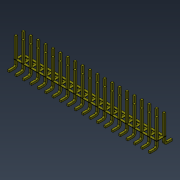
# Autodesk Inventor part: T-1S6-16(-01-20-DV)
Saved by Autodesk Inventor 2022.1 (Build 261234020, 234B)
## iProperties
Created: 2015-08-01
Part Number: T-1S6-16(-01-20-DV)
Catalog Web Link: www.cadenas.de
Description: TSM Series Terminal-TSM Series - (2,54 mm) .100" Surface Mount Terminal .025" Square Post Header
Vendor: SAMTEC
Document SubType Name: Modeling
Designer: PARTuser1
Manufacturer: SAMTEC
Mass: 0.198411 g
Surface Area: 13.9569 cm^2
Volume: 0.198411 cm^3
Density: 1 g/cm^3
Material: Allgemein
Appearance: PSOLRGB-255-255-0
Category: PARTsolutions
Company: SAMTEC
PSOL_IDENT_0: {$CADENAS_DATA\23d-libs\samtec\modelling\tsm\parts\tsm_terminal.prj},210 {VTYP=3D},{NB=T-1S6-16(-01-
PSOL_IDENT_1: 20-DV)},{LINA=T-1S6-16(-01-20-DV)},{NN=TSM Series Terminal},{DATE=20.05.2015 06:36:02},{GEOMDATE=20.
PSOL_IDENT_2: 05.2015 06:36:00},{VERSION=},{LINEID=10},{LINESUBID=-1},{WBVAR=POS,LS,ROW,POLOPT}  {NB=T-1S6-16(-01-
PSOL_IDENT_3: 20-DV)},{LINA=T-1S6-16(-01-20-DV)},{KT=DUMMY},{PN=T-1S6-16},{POS=20},{LS=-01},{LSALG= '-01','-01','-
PSOL_IDENT_4: 02','-02','-03','-03','-04','-04' ,'-05','-05 (Non-standard option -  Please contact SAMTEC)' },{ROW=
PSOL_IDENT_5: -DV},{ROWALG= '-SV','-SV - Single Vertical', '-SH','-SH - Single Horizontal', '-DV' ,'-DV - Double V
PSOL_IDENT_6: ertical' ,'-DV-S' ,'-DV-S - Double Vertical Molded End Shrouds (Non-standard option -  Please contac
PSOL_IDENT_7: t SAMTEC)', '-DH', '-DH - Double Horizontal' ,  '-MT','-MT - Mixed Technology','-EM','-EM - Edge Mou
PSOL_IDENT_8: nt', '-TM','-TM - Triple Mixed Technology'  },{POLOPT=},{POLOPTALG= '','Not Selected','001','001','0
PSOL_IDENT_9: 02','002','003','003','004','004','005','005','006','006','007','007','008','008','009','009','010','
PSOL_IDENT_10: 010','011','011','012','012','013','013','014','014','015','015','016','016','017','017','018','018'
PSOL_IDENT_11: ,'019','019','020','020','021','021','022','022','023','023','024','024','025','025','026','026','02
PSOL_IDENT_12: 7','027','028','028','029','029','030','030','031','031','032','032','033','033','034','034','035','
PSOL_IDENT_13: 035','036','036','037','037','038','038','039','039','040','040' },{POLOPTMAX=480},{POLOPTMAX2='001'
PSOL_IDENT_14: ,'001','002','002','003','003','004','004','005','005','006','006','007','007','008','008','009','00
PSOL_IDENT_15: 9','010','010','011','011','012','012','013','013','014','014','015','015','016','016','017','017','
PSOL_IDENT_16: 018','018','019','019','020','020','021','021','022','022','023','023','024','024','025','025','026'
PSOL_IDENT_17: ,'026','027','027','028','028','029','029','030','030','031','031','032','032','033','033','034','03
PSOL_IDENT_18: 4','035','035','036','036','037','037','038','038','039','039','040','040'},{POLARIZE='001','001','0
PSOL_IDENT_19: 02','002','003','003','004','004','005','005','006','006','007','007','008','008','009','009','010','
PSOL_IDENT_20: 010','011','011','012','012','013','013','014','014','015','015','016','016','017','017','018','018'
PSOL_IDENT_21: ,'019','019','020','020','021','021','022','022','023','023','024','024','025','025','026','026','02
PSOL_IDENT_22: 7','027','028','028','029','029','030','030','031','031','032','032','033','033','034','034','035','
PSOL_IDENT_23: 035','036','036','037','037','038','038','039','039','040','040','041','041','042','042','043','043'
PSOL_IDENT_24: ,'044','044','045','045','046','046','047','047','048','048','049','049','050','050','051','051','05
PSOL_IDENT_25: 2','052','053','053','054','054','055','055','056','056','057','057','058','058','059','059','060','
PSOL_IDENT_26: 060','061','061','062','062','063','063','064','064','065','065','066','066','067','067','068','068'
PSOL_IDENT_27: ,'069','069','070','070','071','071','072','072','073','073','074','074','075','075','076','076','07
PSOL_IDENT_28: 7','077','078','078','079','079','080','080','081','081','082','082','083','083','084','084','085','
PSOL_IDENT_29: 085','086','086','087','087','088','088','089','089','090','090','091','091','092','092','093','093'
PSOL_IDENT_30: ,'094','094','095','095','096','096','097','097','098','098','099','099','100','100','101','101','10
PSOL_IDENT_31: 2','102','103','103','104','104','105','105','106','106','107','107','108','108','109','109','110','
PSOL_IDENT_32: 110','111','111','112','112','113','113','114','114','115','115','116','116','117','117','118','118'
PSOL_IDENT_33: ,'119','119','120','120','121','121','122','122','123','123','124','124','125','125','126','126','12
PSOL_IDENT_34: 7','127','128','128','129','129','130','130','131','131','132','132','133','133','134','134','135','
PSOL_IDENT_35: 135','136','136','137','137','138','138','139','139','140','140','141','141','142','142','143','143'
PSOL_IDENT_36: ,'144','144','145','145','146','146','147','147','148','148','149','149','150','150'},{POLOPTPN=},{P
PSOL_IDENT_37: OLOPTATOF=0},{BSH=0.230},{CSH=0.180},{BSV=0.230},{DMAXSV=0.208},{AEM=0.230},{POLOE=0},{CDHMT=0.230},
PSOL_IDENT_38: {BDVTM=0.23000},{CDV=0.30300},{POLTM=0}
NN: TSM Series Terminal
NT: TSM Series - (2,54 mm) .100" Surface Mount Terminal .025" Square Post Header
NB: T-1S6-16(-01-20-DV)
NBSYN: $PN.($LS.-$POS.$ROW.$POLOPT.)
LINA: T-1S6-16(-01-20-DV)
POS: 20
LS: -01
ROW: -DV - Double Vertical
POLOPT: Not Selected
SUPPLIER: SAMTEC
ARTICLENO: T-1S6-16(-01-20-DV)
BOMINFO: T-1S6-16(-01-20-DV)
CREATOR: CADENAS GmbH
Title: T-1S6-16(-01-20-DV)
Author: Cadenas PARTsolutions
Comments: TSM Series - (2,54 mm) .100" Surface Mount Terminal .025" Square Post Header
Autodesk Inventor part; units mm, degrees
sketch "Sketch_1" plane through (0, 0, 0) normal (1, 0, 0) x (0, 1, 0)
  line L0 (0.635, 2.5781) -> (0, 2.5781)
  line L1 (0, 2.5781) -> (0, 0.6985)
  arc A0 (0, 0.6985) -> (1.016, -0.3175) centre (1.016, 0.6985) ccw
  line L2 (1.016, -0.3175) -> (9.652, -0.3175)
  line L3 (9.652, -0.3175) -> (9.652, 0.3175)
  line L4 (9.652, 0.3175) -> (1.143, 0.3175)
  arc A1 (0.635, 0.8255) -> (1.143, 0.3175) centre (1.143, 0.8255) ccw
  line L5 (0.635, 0.8255) -> (0.635, 2.5781)
  constraints: 12 end point, 4 point on circle, 2 centre point
extrude "Extrusion1" add sketch "Sketch_1" along normal mid plane 48.895
sketch "Sketch_4" plane through (0, 2.54, 0) normal (0, 1, 0) x (1, 0, 0)
  line L0 (-24.4983, 2.9083) -> (-24.4983, -0.3683)
  line L1 (-24.4983, -0.3683) -> (24.4983, -0.3683)
  line L2 (24.4983, -0.3683) -> (24.4983, 2.9083)
  line L3 (24.4983, 2.9083) -> (-24.4983, 2.9083)
  line L4 (21.9583, 2.1717) -> (21.9583, 0.3683)
  line L5 (21.9583, 0.3683) -> (23.7617, 0.3683)
  line L6 (23.7617, 0.3683) -> (23.7617, 2.1717)
  line L7 (23.7617, 2.1717) -> (21.9583, 2.1717)
  line L8 (19.4183, 2.1717) -> (19.4183, 0.3683)
  line L9 (19.4183, 0.3683) -> (21.2217, 0.3683)
  line L10 (21.2217, 0.3683) -> (21.2217, 2.1717)
  line L11 (21.2217, 2.1717) -> (19.4183, 2.1717)
  line L12 (16.8783, 2.1717) -> (16.8783, 0.3683)
  line L13 (16.8783, 0.3683) -> (18.6817, 0.3683)
  line L14 (18.6817, 0.3683) -> (18.6817, 2.1717)
  line L15 (18.6817, 2.1717) -> (16.8783, 2.1717)
  line L16 (14.3383, 2.1717) -> (14.3383, 0.3683)
  line L17 (14.3383, 0.3683) -> (16.1417, 0.3683)
  line L18 (16.1417, 0.3683) -> (16.1417, 2.1717)
  line L19 (16.1417, 2.1717) -> (14.3383, 2.1717)
  line L20 (11.7983, 2.1717) -> (11.7983, 0.3683)
  line L21 (11.7983, 0.3683) -> (13.6017, 0.3683)
  line L22 (13.6017, 0.3683) -> (13.6017, 2.1717)
  line L23 (13.6017, 2.1717) -> (11.7983, 2.1717)
  line L24 (9.2583, 2.1717) -> (9.2583, 0.3683)
  line L25 (9.2583, 0.3683) -> (11.0617, 0.3683)
  line L26 (11.0617, 0.3683) -> (11.0617, 2.1717)
  line L27 (11.0617, 2.1717) -> (9.2583, 2.1717)
  line L28 (6.7183, 2.1717) -> (6.7183, 0.3683)
  line L29 (6.7183, 0.3683) -> (8.5217, 0.3683)
  line L30 (8.5217, 0.3683) -> (8.5217, 2.1717)
  line L31 (8.5217, 2.1717) -> (6.7183, 2.1717)
  line L32 (4.1783, 2.1717) -> (4.1783, 0.3683)
  line L33 (4.1783, 0.3683) -> (5.9817, 0.3683)
  line L34 (5.9817, 0.3683) -> (5.9817, 2.1717)
  line L35 (5.9817, 2.1717) -> (4.1783, 2.1717)
  line L36 (1.6383, 2.1717) -> (1.6383, 0.3683)
  line L37 (1.6383, 0.3683) -> (3.4417, 0.3683)
  line L38 (3.4417, 0.3683) -> (3.4417, 2.1717)
  line L39 (3.4417, 2.1717) -> (1.6383, 2.1717)
  line L40 (-0.9017, 2.1717) -> (-0.9017, 0.3683)
  line L41 (-0.9017, 0.3683) -> (0.9017, 0.3683)
  line L42 (0.9017, 0.3683) -> (0.9017, 2.1717)
  line L43 (0.9017, 2.1717) -> (-0.9017, 2.1717)
  line L44 (-3.4417, 2.1717) -> (-3.4417, 0.3683)
  line L45 (-3.4417, 0.3683) -> (-1.6383, 0.3683)
  line L46 (-1.6383, 0.3683) -> (-1.6383, 2.1717)
  line L47 (-1.6383, 2.1717) -> (-3.4417, 2.1717)
  line L48 (-5.9817, 2.1717) -> (-5.9817, 0.3683)
  line L49 (-5.9817, 0.3683) -> (-4.1783, 0.3683)
  line L50 (-4.1783, 0.3683) -> (-4.1783, 2.1717)
  line L51 (-4.1783, 2.1717) -> (-5.9817, 2.1717)
  line L52 (-8.5217, 2.1717) -> (-8.5217, 0.3683)
  line L53 (-8.5217, 0.3683) -> (-6.7183, 0.3683)
  line L54 (-6.7183, 0.3683) -> (-6.7183, 2.1717)
  line L55 (-6.7183, 2.1717) -> (-8.5217, 2.1717)
  line L56 (-11.0617, 2.1717) -> (-11.0617, 0.3683)
  line L57 (-11.0617, 0.3683) -> (-9.2583, 0.3683)
  line L58 (-9.2583, 0.3683) -> (-9.2583, 2.1717)
  line L59 (-9.2583, 2.1717) -> (-11.0617, 2.1717)
  line L60 (-13.6017, 2.1717) -> (-13.6017, 0.3683)
  line L61 (-13.6017, 0.3683) -> (-11.7983, 0.3683)
  line L62 (-11.7983, 0.3683) -> (-11.7983, 2.1717)
  line L63 (-11.7983, 2.1717) -> (-13.6017, 2.1717)
  line L64 (-16.1417, 2.1717) -> (-16.1417, 0.3683)
  line L65 (-16.1417, 0.3683) -> (-14.3383, 0.3683)
  line L66 (-14.3383, 0.3683) -> (-14.3383, 2.1717)
  line L67 (-14.3383, 2.1717) -> (-16.1417, 2.1717)
  line L68 (-18.6817, 2.1717) -> (-18.6817, 0.3683)
  line L69 (-18.6817, 0.3683) -> (-16.8783, 0.3683)
  line L70 (-16.8783, 0.3683) -> (-16.8783, 2.1717)
  line L71 (-16.8783, 2.1717) -> (-18.6817, 2.1717)
  line L72 (-21.2217, 2.1717) -> (-21.2217, 0.3683)
  line L73 (-21.2217, 0.3683) -> (-19.4183, 0.3683)
  line L74 (-19.4183, 0.3683) -> (-19.4183, 2.1717)
  line L75 (-19.4183, 2.1717) -> (-21.2217, 2.1717)
  line L76 (-23.7617, 2.1717) -> (-23.7617, 0.3683)
  line L77 (-23.7617, 0.3683) -> (-21.9583, 0.3683)
  line L78 (-21.9583, 0.3683) -> (-21.9583, 2.1717)
  line L79 (-21.9583, 2.1717) -> (-23.7617, 2.1717)
  constraints: 160 end point
extrude "Extrusion2" add sketch "Sketch_4" along normal blind 0.127
sketch "Sketch_5" plane through (0, 0, 0) normal (1, 0, 0) x (0, 1, 0)
  arc A0 (1.016, -2.2225) -> (0, -3.2385) centre (1.016, -3.2385) ccw
  line L0 (0, -3.2385) -> (0, -5.1181)
  line L1 (0, -5.1181) -> (0.635, -5.1181)
  line L2 (0.635, -5.1181) -> (0.635, -3.3655)
  arc A1 (1.143, -2.8575) -> (0.635, -3.3655) centre (1.143, -3.3655) ccw
  line L3 (1.143, -2.8575) -> (9.652, -2.8575)
  line L4 (9.652, -2.8575) -> (9.652, -2.2225)
  line L5 (9.652, -2.2225) -> (1.016, -2.2225)
  constraints: 12 end point, 4 point on circle, 2 centre point
extrude "Extrusion3" add sketch "Sketch_5" along normal mid plane 48.895
sketch "Sketch_7" plane through (0, 0, 0) normal (0, 0, 1) x (1, 0, 0)
  line L0 (-23.8125, 18.0594) -> (-23.8125, 2.667)
  line L1 (-23.8125, 2.667) -> (-21.9075, 2.667)
  line L2 (-21.9075, 2.667) -> (-21.9075, 15.3924)
  line L3 (-21.9075, 15.3924) -> (-21.2725, 15.3924)
  line L4 (-21.2725, 15.3924) -> (-21.2725, 2.667)
  line L5 (-21.2725, 2.667) -> (-19.3675, 2.667)
  line L6 (-19.3675, 2.667) -> (-19.3675, 15.3924)
  line L7 (-19.3675, 15.3924) -> (-18.7325, 15.3924)
  line L8 (-18.7325, 15.3924) -> (-18.7325, 2.667)
  line L9 (-18.7325, 2.667) -> (-16.8275, 2.667)
  line L10 (-16.8275, 2.667) -> (-16.8275, 15.3924)
  line L11 (-16.8275, 15.3924) -> (-16.1925, 15.3924)
  line L12 (-16.1925, 15.3924) -> (-16.1925, 2.667)
  line L13 (-16.1925, 2.667) -> (-14.2875, 2.667)
  line L14 (-14.2875, 2.667) -> (-14.2875, 15.3924)
  line L15 (-14.2875, 15.3924) -> (-13.6525, 15.3924)
  line L16 (-13.6525, 15.3924) -> (-13.6525, 2.667)
  line L17 (-13.6525, 2.667) -> (-11.7475, 2.667)
  line L18 (-11.7475, 2.667) -> (-11.7475, 15.3924)
  line L19 (-11.7475, 15.3924) -> (-11.1125, 15.3924)
  line L20 (-11.1125, 15.3924) -> (-11.1125, 2.667)
  line L21 (-11.1125, 2.667) -> (-9.2075, 2.667)
  line L22 (-9.2075, 2.667) -> (-9.2075, 15.3924)
  line L23 (-9.2075, 15.3924) -> (-8.5725, 15.3924)
  line L24 (-8.5725, 15.3924) -> (-8.5725, 2.667)
  line L25 (-8.5725, 2.667) -> (-6.6675, 2.667)
  line L26 (-6.6675, 2.667) -> (-6.6675, 15.3924)
  line L27 (-6.6675, 15.3924) -> (-6.0325, 15.3924)
  line L28 (-6.0325, 15.3924) -> (-6.0325, 2.667)
  line L29 (-6.0325, 2.667) -> (-4.1275, 2.667)
  line L30 (-4.1275, 2.667) -> (-4.1275, 15.3924)
  line L31 (-4.1275, 15.3924) -> (-3.4925, 15.3924)
  line L32 (-3.4925, 15.3924) -> (-3.4925, 2.667)
  line L33 (-3.4925, 2.667) -> (-1.5875, 2.667)
  line L34 (-1.5875, 2.667) -> (-1.5875, 15.3924)
  line L35 (-1.5875, 15.3924) -> (-0.9525, 15.3924)
  line L36 (-0.9525, 15.3924) -> (-0.9525, 2.667)
  line L37 (-0.9525, 2.667) -> (0.9525, 2.667)
  line L38 (0.9525, 2.667) -> (0.9525, 15.3924)
  line L39 (0.9525, 15.3924) -> (1.5875, 15.3924)
  line L40 (1.5875, 15.3924) -> (1.5875, 2.667)
  line L41 (1.5875, 2.667) -> (3.4925, 2.667)
  line L42 (3.4925, 2.667) -> (3.4925, 15.3924)
  line L43 (3.4925, 15.3924) -> (4.1275, 15.3924)
  line L44 (4.1275, 15.3924) -> (4.1275, 2.667)
  line L45 (4.1275, 2.667) -> (6.0325, 2.667)
  line L46 (6.0325, 2.667) -> (6.0325, 15.3924)
  line L47 (6.0325, 15.3924) -> (6.6675, 15.3924)
  line L48 (6.6675, 15.3924) -> (6.6675, 2.667)
  line L49 (6.6675, 2.667) -> (8.5725, 2.667)
  line L50 (8.5725, 2.667) -> (8.5725, 15.3924)
  line L51 (8.5725, 15.3924) -> (9.2075, 15.3924)
  line L52 (9.2075, 15.3924) -> (9.2075, 2.667)
  line L53 (9.2075, 2.667) -> (11.1125, 2.667)
  line L54 (11.1125, 2.667) -> (11.1125, 15.3924)
  line L55 (11.1125, 15.3924) -> (11.7475, 15.3924)
  line L56 (11.7475, 15.3924) -> (11.7475, 2.667)
  line L57 (11.7475, 2.667) -> (13.6525, 2.667)
  line L58 (13.6525, 2.667) -> (13.6525, 15.3924)
  line L59 (13.6525, 15.3924) -> (14.2875, 15.3924)
  line L60 (14.2875, 15.3924) -> (14.2875, 2.667)
  line L61 (14.2875, 2.667) -> (16.1925, 2.667)
  line L62 (16.1925, 2.667) -> (16.1925, 15.3924)
  line L63 (16.1925, 15.3924) -> (16.8275, 15.3924)
  line L64 (16.8275, 15.3924) -> (16.8275, 2.667)
  line L65 (16.8275, 2.667) -> (18.7325, 2.667)
  line L66 (18.7325, 2.667) -> (18.7325, 15.3924)
  line L67 (18.7325, 15.3924) -> (19.3675, 15.3924)
  line L68 (19.3675, 15.3924) -> (19.3675, 2.667)
  line L69 (19.3675, 2.667) -> (21.2725, 2.667)
  line L70 (21.2725, 2.667) -> (21.2725, 15.3924)
  line L71 (21.2725, 15.3924) -> (21.9075, 15.3924)
  line L72 (21.9075, 15.3924) -> (21.9075, 2.667)
  line L73 (21.9075, 2.667) -> (23.8125, 2.667)
  line L74 (23.8125, 2.667) -> (23.8125, 18.0594)
  line L75 (23.8125, 18.0594) -> (-23.8125, 18.0594)
  constraints: 152 end point
extrude "Extrusion4" cut sketch "Sketch_7" along normal mid plane 10.16
sketch "Sketch_8" plane through (0, 0, 0) normal (0, 0, 1) x (1, 0, 0)
  line L0 (-23.8125, -12.8524) -> (23.8125, -12.8524)
  line L1 (23.8125, -12.8524) -> (23.8125, 2.54)
  line L2 (23.8125, 2.54) -> (21.9075, 2.54)
  line L3 (21.9075, 2.54) -> (21.9075, -12.5984)
  line L4 (21.9075, -12.5984) -> (21.2725, -12.5984)
  line L5 (21.2725, -12.5984) -> (21.2725, 2.54)
  line L6 (21.2725, 2.54) -> (19.3675, 2.54)
  line L7 (19.3675, 2.54) -> (19.3675, -12.5984)
  line L8 (19.3675, -12.5984) -> (18.7325, -12.5984)
  line L9 (18.7325, -12.5984) -> (18.7325, 2.54)
  line L10 (18.7325, 2.54) -> (16.8275, 2.54)
  line L11 (16.8275, 2.54) -> (16.8275, -12.5984)
  line L12 (16.8275, -12.5984) -> (16.1925, -12.5984)
  line L13 (16.1925, -12.5984) -> (16.1925, 2.54)
  line L14 (16.1925, 2.54) -> (14.2875, 2.54)
  line L15 (14.2875, 2.54) -> (14.2875, -12.5984)
  line L16 (14.2875, -12.5984) -> (13.6525, -12.5984)
  line L17 (13.6525, -12.5984) -> (13.6525, 2.54)
  line L18 (13.6525, 2.54) -> (11.7475, 2.54)
  line L19 (11.7475, 2.54) -> (11.7475, -12.5984)
  line L20 (11.7475, -12.5984) -> (11.1125, -12.5984)
  line L21 (11.1125, -12.5984) -> (11.1125, 2.54)
  line L22 (11.1125, 2.54) -> (9.2075, 2.54)
  line L23 (9.2075, 2.54) -> (9.2075, -12.5984)
  line L24 (9.2075, -12.5984) -> (8.5725, -12.5984)
  line L25 (8.5725, -12.5984) -> (8.5725, 2.54)
  line L26 (8.5725, 2.54) -> (6.6675, 2.54)
  line L27 (6.6675, 2.54) -> (6.6675, -12.5984)
  line L28 (6.6675, -12.5984) -> (6.0325, -12.5984)
  line L29 (6.0325, -12.5984) -> (6.0325, 2.54)
  line L30 (6.0325, 2.54) -> (4.1275, 2.54)
  line L31 (4.1275, 2.54) -> (4.1275, -12.5984)
  line L32 (4.1275, -12.5984) -> (3.4925, -12.5984)
  line L33 (3.4925, -12.5984) -> (3.4925, 2.54)
  line L34 (3.4925, 2.54) -> (1.5875, 2.54)
  line L35 (1.5875, 2.54) -> (1.5875, -12.5984)
  line L36 (1.5875, -12.5984) -> (0.9525, -12.5984)
  line L37 (0.9525, -12.5984) -> (0.9525, 2.54)
  line L38 (0.9525, 2.54) -> (-0.9525, 2.54)
  line L39 (-0.9525, 2.54) -> (-0.9525, -12.5984)
  line L40 (-0.9525, -12.5984) -> (-1.5875, -12.5984)
  line L41 (-1.5875, -12.5984) -> (-1.5875, 2.54)
  line L42 (-1.5875, 2.54) -> (-3.4925, 2.54)
  line L43 (-3.4925, 2.54) -> (-3.4925, -12.5984)
  line L44 (-3.4925, -12.5984) -> (-4.1275, -12.5984)
  line L45 (-4.1275, -12.5984) -> (-4.1275, 2.54)
  line L46 (-4.1275, 2.54) -> (-6.0325, 2.54)
  line L47 (-6.0325, 2.54) -> (-6.0325, -12.5984)
  line L48 (-6.0325, -12.5984) -> (-6.6675, -12.5984)
  line L49 (-6.6675, -12.5984) -> (-6.6675, 2.54)
  line L50 (-6.6675, 2.54) -> (-8.5725, 2.54)
  line L51 (-8.5725, 2.54) -> (-8.5725, -12.5984)
  line L52 (-8.5725, -12.5984) -> (-9.2075, -12.5984)
  line L53 (-9.2075, -12.5984) -> (-9.2075, 2.54)
  line L54 (-9.2075, 2.54) -> (-11.1125, 2.54)
  line L55 (-11.1125, 2.54) -> (-11.1125, -12.5984)
  line L56 (-11.1125, -12.5984) -> (-11.7475, -12.5984)
  line L57 (-11.7475, -12.5984) -> (-11.7475, 2.54)
  line L58 (-11.7475, 2.54) -> (-13.6525, 2.54)
  line L59 (-13.6525, 2.54) -> (-13.6525, -12.5984)
  line L60 (-13.6525, -12.5984) -> (-14.2875, -12.5984)
  line L61 (-14.2875, -12.5984) -> (-14.2875, 2.54)
  line L62 (-14.2875, 2.54) -> (-16.1925, 2.54)
  line L63 (-16.1925, 2.54) -> (-16.1925, -12.5984)
  line L64 (-16.1925, -12.5984) -> (-16.8275, -12.5984)
  line L65 (-16.8275, -12.5984) -> (-16.8275, 2.54)
  line L66 (-16.8275, 2.54) -> (-18.7325, 2.54)
  line L67 (-18.7325, 2.54) -> (-18.7325, -12.5984)
  line L68 (-18.7325, -12.5984) -> (-19.3675, -12.5984)
  line L69 (-19.3675, -12.5984) -> (-19.3675, 2.54)
  line L70 (-19.3675, 2.54) -> (-21.2725, 2.54)
  line L71 (-21.2725, 2.54) -> (-21.2725, -12.5984)
  line L72 (-21.2725, -12.5984) -> (-21.9075, -12.5984)
  line L73 (-21.9075, -12.5984) -> (-21.9075, 2.54)
  line L74 (-21.9075, 2.54) -> (-23.8125, 2.54)
  line L75 (-23.8125, 2.54) -> (-23.8125, -12.8524)
  constraints: 152 end point
extrude "Extrusion5" cut sketch "Sketch_8" along normal mid plane 15.24
ref_plane "terminal_dv_XY" through (0, 2.54, -1.27) normal (0, 1, 0) x (1, 0, 0)
ref_plane "terminal_dv_YZ" through (0, 2.54, -1.27) normal (1, 0, 0) x (0, 0, -1)
ref_plane "terminal_dv_ZX" through (0, 2.54, -1.27) normal (0, 0, -1) x (0, 1, 0)
body "Solid1"
